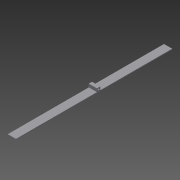
# Autodesk Inventor part: Part2
Saved by Autodesk Inventor 2014 SP1 (Build 180222100, 222)
## iProperties
Created: 2018-05-14
Part Number: Part2
Material: Generic
Document SubType Name: Modeling
Designer: Dadang
Density: 1 g/cm^3
Appearance: Default
Author: Dadang
Autodesk Inventor part; units mm, degrees
ref_plane "YZ Plane" through (0, 0, 0) normal (1, 0, 0) x (0, 1, 0)
ref_plane "XZ Plane" through (0, 0, 0) normal (0, 1, 0) x (-1, 0, 0)
sketch "Sketch1" plane through (0, 0, 0) normal (0, 0, 1) x (1, 0, 0)
  line L0 (0, 0) -> (50, 0)
  line L1 (50, 0) -> (50, 5)
  line L2 (50, 5) -> (0, 5)
  line L3 (0, 5) -> (0, 0)
  dimension "d0" = 50
  dimension "d1" = 5
  constraints: 8 end point, 2 parallel, 1 horizontal, 1 perpendicular
  measures "d0" distance of L2.end L1.end
  measures "d1" distance of L1.end L0.end
extrude "Extrusion1" add sketch "Sketch1" along normal blind 955
ref_plane "Work Plane1" through (0, 0, 0) normal (0, 0, 1) x (1, 0, 0)
sketch "Sketch3" plane through (0, 0, 0) normal (0, 0, 1) x (1, 0, 0)
  line L0 (0, 0) -> (50, 0) projected
  line L1 (0, 5) -> (0, 0) projected
  line L2 (50, 5) -> (0, 5) projected
  line L3 (50, 0) -> (50, 5) projected
  line L4 (0, 5) -> (50, 5) projected
  line L5 (0, 5) -> (0, 25) projected
  line L6 (50, 25) -> (0, 25) projected
  line L7 (50, 5) -> (50, 25) projected
sketch "Sketch5" plane through (0, 5, 0) normal (0, 1, 0) x (1, 0, 0)
  line L0 (50, 0) -> (50, -955) projected
  line L1 (0, -450) -> (0, -460)
  line L2 (0, -460) -> (0, -450)
  line L3 (0, -460) -> (50, -460)
  line L4 (0, 0) -> (0, -955) projected
  line L5 (0, -450) -> (0, -440)
  line L6 (0, -440) -> (50, -440)
  point P0 (50, -450)
  dimension "d22" = 10
  dimension "d27" = 10
  constraints: 10 end point, 4 point on line, 2 perpendicular
  measures "d22" distance of L1.start L1.end
  measures "d27" distance of L1.start L5.end
extrude "Extrusion4" add sketch "Sketch5" along normal blind 20
sketch "Sketch6" plane through (50, 0, 955) normal (1, 0, 0) x (0, 0, -1)
  circle A0 centre (505, 15) radius 5
  dimension "d28" = 10
  constraints: 1 centre point
  measures "d28" diameter of A0
extrude "Extrusion5" cut sketch "Sketch6" against normal blind 50
body "Solid1"
